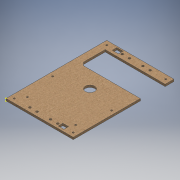
# Autodesk Inventor part: 2枚目kai
Saved by Autodesk Inventor 2018.3 (Build 223284000, 284)
## iProperties
Created: 2018-08-15
Part Number: 2枚目kai
Material: MDF 中密度繊維ボード
Document SubType Name: Modeling
Designer: shun2
Density: 0.8 g/cm^3
Appearance: ダンボール - 段ボール紙
Author: shun2
Autodesk Inventor part; units mm, degrees
ref_plane "YZ Plane" through (0, 0, 0) normal (1, 0, 0) x (0, 1, 0)
ref_plane "XZ Plane" through (0, 0, 0) normal (0, 1, 0) x (-1, 0, 0)
ref_plane "XY Plane" through (0, 0, 0) normal (0, 0, 1) x (1, 0, 0)
sketch "スケッチ3" plane through (0, 0, 0) normal (0, 0, 1) x (1, 0, 0)
  line L0 (129.999999, 177.723921) -> (129.999999, 194.723921)
  line L1 (129.999999, 194.723921) -> (-0.000001, 194.723921)
  line L2 (-0.000001, 0) -> (129.999999, 0)
  circle A0 centre (77.999999, 186.723921) radius 2.15
  circle A1 centre (91.999999, 186.723921) radius 2.15
  circle A2 centre (51.999999, 186.723921) radius 2.15
  circle A3 centre (37.999999, 186.723921) radius 2.15
  circle A4 centre (77.999999, 8) radius 2.15
  circle A5 centre (91.999999, 8) radius 2.15
  circle A6 centre (51.999999, 8) radius 2.15
  circle A7 centre (37.999999, 8) radius 2.15
  line L3 (129.999999, 129.723921) -> (19.999999, 129.723921)
  line L4 (13.999999, 135.723921) -> (13.999999, 177.723921)
  line L5 (13.999999, 177.723921) -> (129.999999, 177.723921)
  line L6 (19.999999, 129.723921) -> (13.999999, 135.723921)
  circle A8 centre (64.999999, 97.36196) radius 8
  circle A9 centre (7.999999, 186.723921) radius 1.6
  circle A10 centre (121.999999, 186.723921) radius 1.6
  circle A11 centre (121.999999, 8) radius 1.6
  circle A12 centre (7.999999, 8) radius 1.6
  circle A13 centre (7.999999, 82) radius 1.6
  circle A14 centre (121.999999, 82) radius 1.6
  line L7 (64.999999, 88.36196) -> (64.999999, 42.36196)
  line L8 (3.399999, 186.723921) -> (12.599999, 186.723921)
  line L9 (7.999999, 182.123921) -> (7.999999, 191.323921)
  line L10 (117.399999, 186.723921) -> (126.599999, 186.723921)
  line L11 (121.999999, 182.123921) -> (121.999999, 191.323921)
  line L12 (117.399999, 8) -> (126.599999, 8)
  line L13 (121.999999, 3.4) -> (121.999999, 12.6)
  line L14 (3.399999, 8) -> (12.599999, 8)
  line L15 (7.999999, 3.4) -> (7.999999, 12.6)
  line L16 (3.399999, 82) -> (12.599999, 82)
  line L17 (7.999999, 77.4) -> (7.999999, 86.6)
  line L18 (126.599999, 82) -> (117.399999, 82)
  line L19 (121.999999, 77.4) -> (121.999999, 86.6)
  circle A15 centre (91.999999, 186.723921) radius 2.15
  circle A16 centre (77.999999, 186.723921) radius 2.15
  circle A17 centre (51.999999, 186.723921) radius 2.15
  circle A18 centre (37.999999, 186.723921) radius 2.15
  circle A19 centre (64.999999, 97.36196) radius 8
  circle A20 centre (91.999999, 8) radius 2.15
  circle A21 centre (77.999999, 8) radius 2.15
  circle A22 centre (51.999999, 8) radius 2.15
  circle A23 centre (37.999999, 8) radius 2.15
  circle A24 centre (7.999999, 8) radius 1.6
  circle A25 centre (121.999999, 8) radius 1.6
  circle A26 centre (121.999999, 82) radius 1.6
  circle A27 centre (121.999999, 186.723921) radius 1.6
  circle A28 centre (7.999999, 186.723921) radius 1.6
  circle A29 centre (7.999999, 82) radius 1.6
  line L20 (-0.000001, 0) -> (129.999999, 0)
  line L21 (129.999999, 177.723921) -> (129.999999, 194.723921)
  line L22 (129.999999, 194.723921) -> (-0.000001, 194.723921)
  line L23 (129.999999, 177.723921) -> (13.999999, 177.723921)
  line L24 (13.999999, 177.723921) -> (13.999999, 135.723921)
  line L25 (13.999999, 135.723921) -> (19.999999, 129.723921)
  line L26 (-0.000001, 194.723921) -> (-0.000001, 119.36196)
  line L27 (-0.000001, 86.6) -> (-0.000001, 0)
  line L28 (-0.000001, 194.723921) -> (-0.000001, 119.36196)
  line L29 (-0.000001, 86.6) -> (-0.000001, 0)
  line L30 (129.999999, 0) -> (129.999999, 86.6)
  line L31 (129.999999, 125.36196) -> (129.999999, 129.723921)
  line L32 (129.999999, 0) -> (129.999999, 86.6)
  line L33 (129.999999, 125.36196) -> (129.999999, 129.723921)
  circle A30 centre (18.296419, 23) radius 1.6
  circle A31 centre (111.703579, 23) radius 1.6
  line L34 (-0.000001, 119.36196) -> (-0.000001, 86.6)
  line L35 (129.999999, 86.6) -> (129.999999, 125.36196)
  point P0 (0, 0)
  point P1 (0, 0)
  constraints: 72 end point, 32 centre point, 15 coincident, 9 concentric, 6 collinear, 3 perpendicular, 3 vertical, 1 parallel
sketch "スケッチ4" plane through (0, 0, 0) normal (0, 0, 1) x (1, 0, 0)
  point P0 (0, 0)
extrude "押し出し1" add sketch "スケッチ3" along normal blind 4 contours L5 L4 L6 L3 L31 L35 L30 L2 L27 L34 L26 L1 L0 | A30 | A31
sketch "スケッチ5" plane through (0, 0, 4) normal (0, 0, 1) x (1, 0, 0)
  line L0 (-10, 0) -> (140, 0)
  arc A0 (140, -0.0003) -> (140, 0.0003) centre (140, 0) ccw
  arc A1 (-10, 0.0003) -> (-10, -0.0003) centre (-10, 0) ccw
  line L1 (140, 0) -> (140, 194.7239)
  arc A2 (140.0002, 194.7239) -> (139.9998, 194.7239) centre (140, 194.7239) ccw
  arc A3 (139.9998, 0) -> (140.0002, 0) centre (140, 0) ccw
  line L2 (140, 194.7239) -> (-10, 194.7239)
  arc A4 (-10, 194.7242) -> (-10, 194.7237) centre (-10, 194.72395) ccw
  arc A5 (140, 194.7237) -> (140, 194.7242) centre (140, 194.72395) ccw
  arc A6 (-10.0004, 0) -> (-10, 0) centre (-10.0002, 0) ccw
  arc A7 (-9.9996, 194.7239) -> (-10, 194.7239) centre (-9.9998, 194.7239) ccw
  arc A8 (65, 88.362) -> (65, 106.362) centre (65, 97.362) ccw
  arc A9 (65, 106.362) -> (65, 88.362) centre (65, 97.362) ccw
  arc A10 (65, 158.7239) -> (65, 176.7239) centre (65, 167.7239) ccw
  arc A11 (65, 176.7239) -> (65, 158.7239) centre (65, 167.7239) ccw
  line L3 (125.6971, 165.1236) -> (118.0771, 165.1236)
  line L4 (115.5371, 165.1236) -> (115.5371, 160.0436)
  line L5 (121.66, 165.205) -> (120.39, 165.205)
  arc A12 (121.66, 165.1669) -> (121.66, 165.2431) centre (121.66, 165.205) ccw
  line L6 (81.02, 174.095) -> (85.719, 174.095)
  arc A13 (81.02, 174.1331) -> (81.02, 174.0569) centre (81.02, 174.095) ccw
  line L7 (81.02, 174.095) -> (81.02, 165.205)
  arc A14 (80.9819, 165.205) -> (81.0581, 165.205) centre (81.02, 165.205) ccw
  arc A15 (81.0581, 174.095) -> (80.9819, 174.095) centre (81.02, 174.095) ccw
  line L8 (121.66, 165.205) -> (121.66, 174.095)
  arc A16 (121.6981, 174.095) -> (121.6219, 174.095) centre (121.66, 174.095) ccw
  arc A17 (121.6219, 165.205) -> (121.6981, 165.205) centre (121.66, 165.205) ccw
  line L9 (82.29, 165.205) -> (81.02, 165.205)
  arc A18 (81.02, 165.2431) -> (81.02, 165.1669) centre (81.02, 165.205) ccw
  line L10 (121.66, 174.095) -> (117.342, 174.095)
  arc A19 (121.66, 174.0569) -> (121.66, 174.1331) centre (121.66, 174.095) ccw
  line L11 (52.85, 166.325) -> (48.151, 166.325)
  arc A20 (52.85, 166.2869) -> (52.85, 166.3631) centre (52.85, 166.325) ccw
  line L12 (52.85, 166.325) -> (52.85, 175.215)
  arc A21 (52.8881, 175.215) -> (52.8119, 175.215) centre (52.85, 175.215) ccw
  arc A22 (52.8119, 166.325) -> (52.8881, 166.325) centre (52.85, 166.325) ccw
  line L13 (51.58, 175.215) -> (52.85, 175.215)
  arc A23 (52.85, 175.1769) -> (52.85, 175.2531) centre (52.85, 175.215) ccw
  arc A24 (72.9742, 175.4632) -> (72.9742, 175.768) centre (72.9742, 175.6156) ccw
  arc A25 (72.9742, 175.768) -> (72.9742, 175.4632) centre (72.9742, 175.6156) ccw
  arc A26 (72.9742, 175.4632) -> (72.9742, 175.768) centre (72.9742, 175.6156) ccw
  arc A27 (72.9742, 175.768) -> (72.9742, 175.4632) centre (72.9742, 175.6156) ccw
  arc A28 (86.106, 110.5662) -> (86.106, 110.871) centre (86.106, 110.7186) ccw
  arc A29 (86.106, 110.871) -> (86.106, 110.5662) centre (86.106, 110.7186) ccw
  arc A30 (86.106, 110.5662) -> (86.106, 110.871) centre (86.106, 110.7186) ccw
  arc A31 (86.106, 110.871) -> (86.106, 110.5662) centre (86.106, 110.7186) ccw
  line L14 (80.9819, 174.095) -> (121.6981, 174.095)
  line L15 (121.6981, 174.095) -> (121.6981, 165.205)
  line L16 (121.6981, 165.205) -> (80.9819, 165.205)
  line L17 (80.9819, 165.205) -> (80.9819, 174.095)
  line L18 (52.8, 176.585002) -> (11.364013, 176.585002)
  line L19 (11.364013, 176.585002) -> (11.364013, 165.1236)
  line L20 (11.364013, 165.1236) -> (52.8, 165.1236)
  line L21 (52.8, 165.1236) -> (52.8, 176.585002)
  line L22 (-10, 194.7239) -> (-10, 0)
  line L23 (21.97, 192.403451) -> (33.97, 192.403451)
  line L24 (33.97, 192.403451) -> (33.97, 183.403451)
  line L25 (33.97, 183.403451) -> (21.97, 183.403451)
  line L26 (21.97, 183.403451) -> (21.97, 192.403451)
  line L27 (0, 0) -> (129.999999, 0)
  line L28 (96.51585, 13.395653) -> (107.51585, 13.395653)
  line L29 (107.51585, 13.395653) -> (107.51585, 4.395653)
  line L30 (107.51585, 4.395653) -> (96.51585, 4.395653)
  line L31 (96.51585, 4.395653) -> (96.51585, 13.395653)
  circle A32 centre (65, 97.362) radius 9
  point P0 (71.80055, 0)
  constraints: 64 point on circle, 62 end point, 33 centre point, 8 parallel, 4 horizontal, 4 perpendicular, 1 coincident, 1 point on line, 1 vertical
sketch "スケッチ5 outline for 押し出し2" plane through (0, 0, 4) normal (0, 0, 1) x (1, 0, 0)
  line L0 (96.51585, 13.395653) -> (107.51585, 13.395653)
  line L1 (107.51585, 13.395653) -> (107.51585, 4.395653)
  line L2 (107.51585, 4.395653) -> (96.51585, 4.395653)
  line L3 (96.51585, 4.395653) -> (96.51585, 13.395653)
  line L4 (21.97, 192.403451) -> (33.97, 192.403451)
  line L5 (33.97, 192.403451) -> (33.97, 183.403451)
  line L6 (33.97, 183.403451) -> (21.97, 183.403451)
  line L7 (21.97, 183.403451) -> (21.97, 192.403451)
  circle A0 centre (65, 97.362) radius 9
  line L8 (121.6981, 165.205) -> (121.6981, 174.095)
  line L9 (80.9819, 165.205) -> (121.6981, 165.205)
  line L10 (80.9819, 174.095) -> (80.9819, 165.205)
  line L11 (121.6981, 174.095) -> (80.9819, 174.095)
extrude "押し出し2" cut sketch "スケッチ5 outline for 押し出し2" against normal blind 10
sketch "スケッチ7" plane through (0, 0, 4) normal (0, 0, 1) x (1, 0, 0)
  point P0 (0, 0)
sketch "スケッチ8" plane through (0, 0, 4) normal (0, 0, 1) x (1, 0, 0)
  circle A0 centre (18.296419, 23) radius 1.6
  circle A1 centre (111.703579, 23) radius 1.6
  point P0 (0, 0)
  constraints: 2 centre point
extrude "押し出し5" cut sketch "スケッチ8" against normal blind 4
